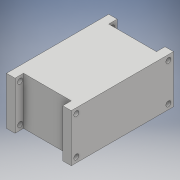
# Autodesk Inventor part: upperarm
Saved by Autodesk Inventor 2018 (Build 220112000, 112)
## iProperties
Created: 2020-09-07
Part Number: upperarm
Material: 일반
Document SubType Name: Modeling
Designer: j3jjj
Density: 1 g/cm^3
Appearance: 기본값
Author: j3jjj
Autodesk Inventor part; units mm, degrees
ref_plane "YZ Plane" through (0, 0, 0) normal (1, 0, 0) x (0, 1, 0)
ref_plane "XZ Plane" through (0, 0, 0) normal (0, 1, 0) x (-1, 0, 0)
ref_plane "XY Plane" through (0, 0, 0) normal (0, 0, 1) x (1, 0, 0)
sketch "스케치1" plane through (0, 0, 0) normal (0, 1, 0) x (-1, 0, 0)
  line L0 (18, -14) -> (-20, -14)
  line L1 (-20, -14) -> (-20, 14)
  line L2 (-20, 14) -> (18, 14)
  line L3 (18, 14) -> (18, -14)
  point P0 (0, 0)
  dimension "d0" = 28
  dimension "d1" = 14
  dimension "d2" = 38
  dimension "d3" = 18
  constraints: 8 end point, 2 parallel, 1 horizontal, 1 perpendicular
  measures "d0" distance between parallel lines of L0 L2
  measures "d1" distance from line of point (0, 0) L2
  measures "d2" distance between parallel lines of L1 L3
  measures "d3" distance from line of point (0, 0) L3
extrude "돌출1" add sketch "스케치1" along normal blind 50
sketch "스케치2" plane through (0, 50, 0) normal (0, 1, 0) x (1, 0, 0)
  line L0 (20, 14) -> (-18, 14) projected
  line L1 (-18, -14) -> (20, -14) projected
  line L2 (-18, 14) -> (-13.01, 14)
  line L3 (-13.01, 14) -> (-13.01, -14)
  line L4 (-13.01, -14) -> (-18, -14)
  line L5 (-18, -14) -> (-18, 14)
  line L6 (20, -14) -> (15.01, -14)
  line L7 (15.01, -14) -> (15.01, 14)
  line L8 (15.01, 14) -> (20, 14)
  line L9 (20, 14) -> (20, -14)
  point P0 (0, 0)
  dimension "d6" = 4.99
  dimension "d7" = 4.99
  constraints: 16 end point, 4 parallel, 2 horizontal, 2 perpendicular, 2 point on line
  measures "d6" distance between parallel lines of L3 L5
  measures "d7" distance between parallel lines of L9 L7
extrude "돌출2" add sketch "스케치2" along normal blind 5 contours L9 L1 L7 L0 | L3 L1 L5 L0
sketch "스케치4" plane through (20, 0, 14) normal (1, 0, 0) x (0, 0, -1)
  circle A0 centre (3, 52) radius 1.5
  circle A1 centre (25, 52) radius 1.5
  line L0 (0, 55) -> (28, 55) projected
  line L1 (28, 0) -> (28, 55) projected
  line L2 (0, 0) -> (0, 55) projected
  point P0 (14, 0)
  dimension "d24" = 3
  dimension "d25" = 3
  dimension "d26" = 3
  dimension "d27" = 3
  dimension "d28" = 3
  dimension "d29" = 3
  constraints: 2 centre point
  measures "d24" diameter of A1
  measures "d25" diameter of A0
  measures "d26" distance from line of A0.centre L0
  measures "d27" distance from line of A1.centre L0
  measures "d28" distance from line of L1 A1.centre
  measures "d29" distance from line of L2 A0.centre
extrude "돌출4" cut sketch "스케치4" against normal blind 80
sketch "스케치5" plane through (0, 0, 0) normal (0, -1, 0) x (1, 0, 0)
  line L0 (20, -14) -> (20, 14) projected
  line L1 (-18, -14) -> (20, -14) projected
  line L2 (20, 14) -> (15.01, 14)
  line L3 (15.01, 14) -> (15.01, -14)
  line L4 (15.01, -14) -> (20, -14)
  line L5 (20, -14) -> (20, 14)
  line L6 (-18, 14) -> (-13.01, 14)
  line L7 (-13.01, 14) -> (-13.01, -14)
  line L8 (-13.01, -14) -> (-18, -14)
  line L9 (-18, -14) -> (-18, 14)
  point P0 (0, 0)
  dimension "d32" = 4.99
  dimension "d33" = 4.99
  constraints: 16 end point, 4 parallel, 3 point on line, 2 horizontal, 2 perpendicular
  measures "d32" distance between parallel lines of L3 L0
  measures "d33" distance between parallel lines of L9 L7
extrude "돌출5" add sketch "스케치5" along normal blind 5
sketch "스케치6" plane through (20, 55, 14) normal (1, 0, 0) x (0, 0, -1)
  circle A0 centre (25, -57) radius 1.5
  circle A1 centre (3, -57) radius 1.5
  line L0 (28, -60) -> (0, -60) projected
  line L1 (28, 0) -> (28, -60) projected
  line L2 (0, 0) -> (0, -60) projected
  point P0 (14, -55)
  dimension "d36" = 3
  dimension "d37" = 3
  dimension "d38" = 3
  dimension "d39" = 3
  dimension "d40" = 3
  dimension "d41" = 3
  constraints: 2 centre point
  measures "d36" diameter of A0
  measures "d37" diameter of A1
  measures "d38" distance from line of L0 A0.centre
  measures "d39" distance from line of L1 A0.centre
  measures "d40" distance from line of L0 A1.centre
  measures "d41" distance from line of L2 A1.centre
extrude "돌출6" cut sketch "스케치6" against normal blind 80
